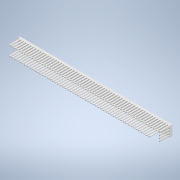
# Autodesk Inventor part: ДИ 00.00.12
Saved by Autodesk Inventor 2021.2 (Build 252289000, 289)
## iProperties
Created: 2021-10-12
Part Number: ДИ 00.00.12
Material: Типовые
Document SubType Name: Modeling
Designer: Surflay
Density: 1 g/cm^3
Appearance: По умолчанию
Author: Surflay
Autodesk Inventor part; units mm, degrees
ref_plane "YZ Plane" through (0, 0, 0) normal (1, 0, 0) x (0, 1, 0)
ref_plane "XZ Plane" through (0, 0, 0) normal (0, 1, 0) x (-1, 0, 0)
sketch "Эскиз1" plane through (0, 0, 0) normal (0, 0, 1) x (1, 0, 0)
  line L0 (45, 39.0097) -> (-45, 39.0097) projected
  line L1 (-45, 39.0097) -> (-45, -39.0097) projected
  line L2 (-45, -39.0097) -> (45, -39.0097) projected
  line L3 (45, -39.0097) -> (45, 39.0097) projected
  line L4 (-35, 36.0097) -> (25, 36.0097)
  line L5 (25, 36.0097) -> (25, 32.0097)
  line L6 (21, 32.0097) -> (-35, 32.0097)
  line L7 (-35, 32.0097) -> (-35, 36.0097)
  line L8 (20.3207, 36.0097) -> (25, 36.0097)
  line L9 (25, 36.0097) -> (25, -28.5789)
  line L10 (25, -28.5789) -> (21, -28.5789)
  line L11 (21, -28.5789) -> (21, 32.0097)
  point P0 (0, 0)
  dimension "d0" = 4
  dimension "d1" = 10
  dimension "d2" = 3
  dimension "d3" = 4
  dimension "d4" = 20
  dimension "d5" = 4
  constraints: 16 end point, 4 parallel, 2 horizontal, 2 perpendicular, 1 point on line
  measures "d0" distance of L4.end L5.end
  measures "d1" distance between parallel lines of L1 L7
  measures "d2" distance between parallel lines of L0 L4
  measures "d3" distance of L9.end L10.end
  measures "d4" distance between parallel lines of L3 L5
  measures "d5" distance between parallel lines of L4 L6
extrude "Выдавливание1" add sketch "Эскиз1" along normal blind 1 contours L4 L5 L9 L10 L11 L6 L7
sketch "Эскиз2" plane through (0, 0, 1) normal (0, 0, 1) x (1, 0, 0)
  line L0 (-35, 36.0097) -> (-35, 32.0097) projected
  line L1 (25, 36.0097) -> (-35, 36.0097) projected
  line L2 (-35, 32.0097) -> (21, 32.0097) projected
  line L3 (21, 32.0097) -> (21, -28.5789) projected
  line L4 (25, -28.5789) -> (25, 36.0097) projected
  line L5 (21, -28.5789) -> (25, -28.5789) projected
  line L6 (-35, 32.3097) -> (21, 32.3097)
  line L7 (21, 32.3097) -> (21, 32.0097)
  line L8 (21, 32.0097) -> (-35, 32.0097)
  line L9 (-35, 32.0097) -> (-35, 32.3097)
  line L10 (21, 32.3097) -> (21.3, 32.3097)
  line L11 (21.3, 32.3097) -> (21.3, -28.5789)
  line L12 (21.3, -28.5789) -> (21, -28.5789)
  line L13 (21, -28.5789) -> (21, 32.3097)
  line L14 (-35, 36.0097) -> (25, 36.0097)
  line L15 (25, 36.0097) -> (25, 35.7097)
  line L16 (25, 35.7097) -> (-35, 35.7097)
  line L17 (-35, 35.7097) -> (-35, 36.0097)
  line L18 (24.7, 36.0097) -> (25, 36.0097)
  line L19 (25, 36.0097) -> (25, -28.5789)
  line L20 (25, -28.5789) -> (24.7, -28.5789)
  line L21 (24.7, -28.5789) -> (24.7, 36.0097)
  point P0 (0, 0)
  point P1 (24.7, 35.7097)
  dimension "d8" = 0.3
  dimension "d9" = 0.3
  dimension "d10" = 0.3
  dimension "d11" = 0.3
  constraints: 32 end point, 8 parallel, 4 horizontal, 4 perpendicular, 4 point on line
  measures "d8" distance between parallel lines of L2 L6
  measures "d9" distance between parallel lines of L3 L11
  measures "d10" distance between parallel lines of L16 L1
  measures "d11" distance between parallel lines of L21 L4
extrude "Выдавливание2" add sketch "Эскиз2" along normal blind 4 contours L1 L21 L16 L0 | L1 L4 L16 L21 | L6 L7 L2 L0 | L16 L4 L5 L21 | L10 L11 L5 L3 L7
sketch "Эскиз3" plane through (21, -28.5789, 0) normal (-1, 0, 0) x (0, 0, 1)
  line L0 (1, 60.8886) -> (1, 0) construction
  line L1 (5, 0) -> (5, 60.8886) construction
  line L2 (5, 0) -> (1, 0) construction
  line L3 (1, 0) -> (1, 0.5) construction
  line L4 (1, 0.5) -> (5, 0.5)
  line L5 (5, 0.5) -> (5, 0) construction
  line L6 (5, 0.5) -> (1, 0.5)
  line L7 (1, 0.5) -> (1, 1)
  line L8 (1, 1) -> (5, 1)
  line L9 (5, 1) -> (5, 0.5)
  point P0 (0, 28.5789)
  point P1 (1, 0.75)
  point P2 (1, 0.5)
  dimension "d14" = 0.5
  dimension "d15" = 0.5
  constraints: 16 end point, 4 parallel, 2 horizontal, 2 perpendicular, 2 point on line, 1 midpoint
  measures "d14" distance of L2.end L3.end
  measures "d15" distance of L6.end L7.end
extrude "Выдавливание3" cut sketch "Эскиз3" against normal through all
pattern_linear "Прямоуг.массив1" count 64 spacing 1 along (0, 1, 0) of "Выдавливание3"
sketch "Эскиз4" plane through (-35, 36.0097, 0) normal (0, 1, 0) x (1, 0, 0)
  line L0 (60, 0) -> (60, -5) projected
  line L1 (59.7, -1) -> (0, -1) projected
  line L2 (60, -5) -> (60, -1) projected
  line L3 (60, -5) -> (59.5, -5)
  line L4 (59.5, -5) -> (59.5, -1)
  line L5 (59.5, -1) -> (60, -1)
  line L6 (60, -1) -> (60, -5)
  line L7 (60, -5) -> (0, -5) projected
  line L8 (59.5, -1) -> (59, -1)
  line L9 (59, -1) -> (59, -5)
  line L10 (59, -5) -> (59.5, -5)
  line L11 (59.5, -5) -> (59.5, -1)
  point P0 (35, 0)
  dimension "d21" = 0.5
  dimension "d22" = 0.5
  constraints: 16 end point, 4 parallel, 2 horizontal, 2 perpendicular, 2 point on line
  measures "d21" distance of L4.end L5.end
  measures "d22" distance of L10.end L9.end
extrude "Выдавливание4" cut sketch "Эскиз4" against normal blind 4 contours L7 L9 L1 L4
pattern_linear "Прямоуг.массив2" count 60 spacing 1 along (-1, 0, 0) of "Выдавливание4"
sketch "Эскиз5" plane through (0, 0, 5) normal (0, 0, 1) x (1, 0, 0)
  line L0 (18.5, 32.0097) -> (19, 32.0097) projected
  line L1 (18.5, 32.0097) -> (28.6813, 32.0097)
  line L2 (28.6813, 32.0097) -> (28.6813, -29.3542)
  line L3 (28.6813, -29.3542) -> (18.5, -29.3542)
  line L4 (18.5, -29.3542) -> (18.5, 32.0097)
  point P0 (0, 0)
  constraints: 8 end point, 2 parallel, 1 horizontal, 1 perpendicular
ref_plane "РабПлоскость1" through (-45, -39.0097, 0) normal (0, 0, 1) x (1, 0, 0)
extrude "Выдавливание5" cut sketch "Эскиз5" against normal up to surface (5 mm away)
